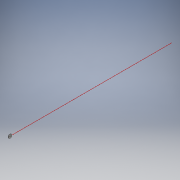
# Autodesk Inventor part: Hook Whip
Saved by Autodesk Inventor 2016 (Build 200138000, 138)
## iProperties
Created: 2016-01-19
Part Number: Hook Whip
Material: Generic
Document SubType Name: Modeling
Designer: TimB
Density: 1 g/cm^3
Appearance: Default
Author: TimB
Autodesk Inventor part; units mm, degrees
ref_plane "YZ Plane" through (0, 0, 0) normal (1, 0, 0) x (0, 1, 0)
ref_plane "XZ Plane" through (0, 0, 0) normal (0, 1, 0) x (-1, 0, 0)
ref_plane "XY Plane" through (0, 0, 0) normal (0, 0, 1) x (1, 0, 0)
sketch "Sketch1" plane through (0, 0, 0) normal (0, 1, 0) x (-1, 0, 0)
  circle A0 centre (0, 0) radius 1
  dimension "d0" = 2
  constraints: 1 centre point, 1 coincident
  measures "d0" diameter of A0
extrude "Extrusion1" add sketch "Sketch1" along normal blind 1200
sketch "Sketch2" plane through (0, 0, 0) normal (0, -1, 0) x (1, 0, 0)
  line L0 (-1, -12.5) -> (1, -12.5)
  line L1 (1, -12.5) -> (1, 12.5)
  line L2 (1, 12.5) -> (-1, 12.5)
  line L3 (-1, 12.5) -> (-1, -12.5)
  line L4 (-1, -12.5) -> (1, 12.5) construction
  line L5 (1, -12.5) -> (-1, 12.5) construction
  point P0 (0, 0)
  dimension "d3" = 2
  dimension "d4" = 25
  constraints: 12 end point, 2 midpoint, 2 parallel, 1 horizontal, 1 perpendicular
  measures "d3" distance of L2.end L1.end
  measures "d4" distance of L1.end L0.end
extrude "Extrusion2" add sketch "Sketch2" against normal blind 25
fillet "Fillet1" radius 10 4 edges at (0, 25, 12.5) (0, 25, -12.5) (0, 0, 12.5) (0, 0, -12.5)
sketch "Sketch3" plane through (-1, 0, -2.5) normal (-1, 0, 0) x (0, 0, 1)
  circle A0 centre (2.5, 12.5) radius 3
  point P0 (2.5, 0)
  dimension "d8" = 6
  constraints: 1 centre point
  measures "d8" diameter of A0
hole "Hole1" at (-1, 12.5, 0) direction (1, 0, 0) diameter 6 end through all
body "Solid1"
